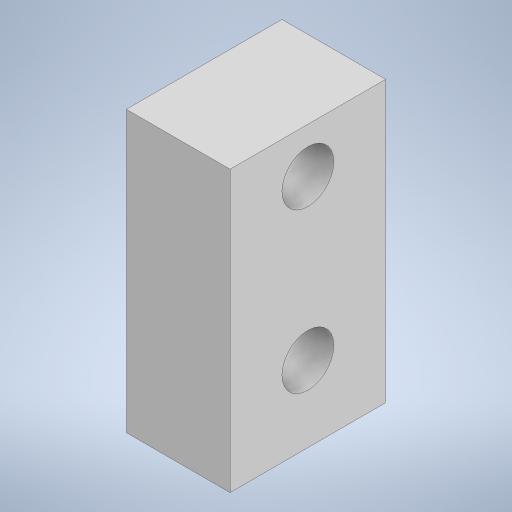
# Autodesk Inventor part: Part2
Saved by Autodesk Inventor 2024 (Build 280153000, 153)
## iProperties
Created: 2024-02-24
Part Number: Part2
Material: Generic
Document SubType Name: Modeling
Designer: anart
Density: 1 g/cm^3
Appearance: Default
Author: anart
Autodesk Inventor part; units mm, degrees
ref_plane "YZ Plane" through (0, 0, 0) normal (1, 0, 0) x (0, 1, 0)
ref_plane "XZ Plane" through (0, 0, 0) normal (0, 1, 0) x (-1, 0, 0)
ref_plane "XY Plane" through (0, 0, 0) normal (0, 0, 1) x (1, 0, 0)
sketch "Sketch1" plane through (0, 0, 0) normal (1, 0, 0) x (0, 1, 0)
  line L0 (0, 0) -> (27, 0)
  line L1 (27, 0) -> (27, 15)
  line L2 (27, 15) -> (0, 15)
  line L3 (0, 15) -> (0, 0)
  dimension "d0" = 27
  dimension "d1" = 15
  constraints: 8 end point, 2 parallel, 1 horizontal, 1 perpendicular
  measures "d0" distance of L2.end L1.end
  measures "d1" distance of L1.end L0.end
extrude "Extrusion1" add sketch "Sketch1" along normal blind 10
sketch "Sketch2" plane through (10, 0, 0) normal (1, 0, 0) x (0, 0, -1)
  line L0 (0, 27) -> (-15, 27) projected
  line L1 (-7.5, 27) -> (-7.5, 0)
  line L2 (-15, 0) -> (0, 0) projected
  line L3 (-10.4795, 25.2) -> (-4.5199, 25.2)
  circle A0 centre (-7.5, 22.6329) radius 2.5
  line L4 (-10.4795, 10) -> (-5, 10)
  circle A1 centre (-7.5, 7.2988) radius 2.5
  dimension "d4" = 1.8
  dimension "d5" = 5
  dimension "d6" = 17
  dimension "d7" = 5
  constraints: 6 end point, 2 centre point, 2 horizontal, 2 midpoint
  measures "d4" distance between parallel lines of L0 L3
  measures "d5" diameter of A0
  measures "d6" distance between parallel lines of L0 L4
  measures "d7" diameter of A1
extrude "Extrusion2" cut sketch "Sketch2" against normal blind 10
sketch "Sketch3" plane through (10, 0, 0) normal (1, 0, 0) x (0, 0, -1)
  point P0 (0, 0)
body "Solid1"
